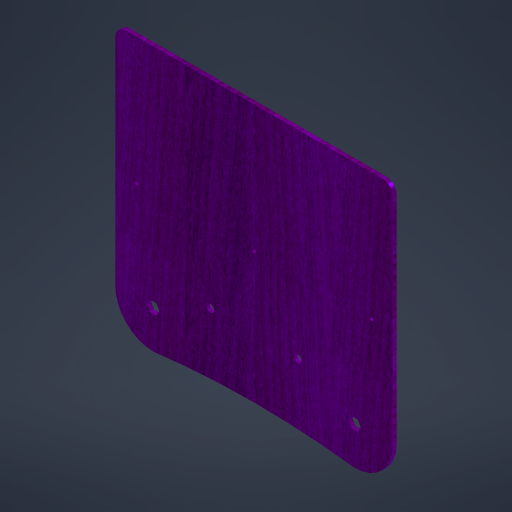
# Autodesk Inventor part: FTC Outside Panels
Saved by Autodesk Inventor 2024.2 (Build 282272000, 272)
## iProperties
Created: 2022-09-22
Part Number: FTC Outside Panels
Material: Wood (Oak)
Document SubType Name: Modeling
Designer: Jason
Density: 0.76 g/cm^3
Appearance: White Oak - Natural Medium Gloss
Author: Jason
Autodesk Inventor part; units mm, degrees
ref_plane "YZ Plane" through (0, 0, 0) normal (1, 0, 0) x (0, 1, 0)
ref_plane "XZ Plane" through (0, 0, 0) normal (0, 1, 0) x (-1, 0, 0)
ref_plane "XY Plane" through (0, 0, 0) normal (0, 0, 1) x (1, 0, 0)
sketch "Sketch1" plane through (0, 0, 0) normal (0, 0, 1) x (1, 0, 0)
  line L0 (0, 0) -> (333.375, 0)
  line L1 (333.375, 0) -> (333.375, 304.8)
  line L2 (320.675, 317.5) -> (12.7, 317.5)
  line L3 (0, 304.8) -> (0, 0)
  circle A0 centre (45.72, 45.72) radius 45.72
  circle A1 centre (287.655, 45.72) radius 45.72
  line L4 (166.6875, 0) -> (166.6875, 7.62)
  arc A2 (287.655, 0) -> (45.72, 0) centre (166.6875, -956.3695) ccw
  arc A3 (12.7, 317.5) -> (0, 304.8) centre (12.7, 304.8) ccw
  arc A4 (333.375, 304.8) -> (320.675, 317.5) centre (320.675, 304.8) ccw
  circle A5 centre (45.72, 45.72) radius 2.413
  circle A6 centre (287.655, 45.72) radius 2.413
  circle A7 centre (25.4, 165.1) radius 2.413
  circle A8 centre (307.975, 165.1) radius 2.413
  line L5 (25.4, 165.1) -> (307.975, 165.1)
  circle A9 centre (166.6875, 165.1) radius 2.413
  line L6 (114.0968, 95.337) -> (114.0968, 63.3371)
  line L7 (114.0968, 45.72) -> (114.0968, 63.3371)
  circle A10 centre (114.1277, 79.3382) radius 4.699
  ellipse E0 centre (114.0968, 63.3371) end of major axis (114.0894, 65.3371) minor radius 2
  line L8 (219.2782, 45.72) -> (219.2782, 63.3371)
  ellipse E1 centre (219.2782, 63.3371) end of major axis (219.2708, 65.3371) minor radius 2
  line L9 (219.2782, 95.3392) -> (219.2782, 63.3371)
  circle A11 centre (219.3091, 79.3382) radius 4.699
  line L10 (45.72, 45.72) -> (114.0968, 45.72)
  line L11 (287.655, 45.72) -> (219.2782, 45.72)
  ellipse E2 centre (235.2526, 141.4087) end of major axis (235.2552, 140.0562) minor radius 1.3525
  ellipse E3 centre (203.2527, 141.3472) end of major axis (203.2553, 139.9947) minor radius 1.3525
  ellipse E4 centre (219.2782, 95.3392) end of major axis (219.2743, 97.3392) minor radius 2
  ellipse E5 centre (219.2782, 95.3392) end of major axis (219.2743, 97.3392) minor radius 2
  ellipse E6 centre (130.4933, 141.0351) end of major axis (130.4959, 139.6826) minor radius 1.3525
  ellipse E7 centre (98.4934, 140.9736) end of major axis (98.496, 139.621) minor radius 1.3525
  ellipse E8 centre (114.0968, 95.337) end of major axis (114.0929, 97.337) minor radius 2
  ellipse E9 centre (114.0968, 95.337) end of major axis (114.0929, 97.337) minor radius 2
  line L12 (49.3862, 39.37) -> (53.0523, 45.72)
  line L13 (49.3862, 52.07) -> (53.0523, 45.72)
  line L14 (42.0538, 39.37) -> (49.3862, 39.37)
  line L15 (42.0538, 52.07) -> (49.3862, 52.07)
  line L16 (42.0538, 52.07) -> (38.3877, 45.72)
  line L17 (38.3877, 45.72) -> (42.0538, 39.37)
  line L18 (291.1818, 39.37) -> (294.848, 45.72)
  line L19 (291.1818, 52.07) -> (294.848, 45.72)
  line L20 (283.8495, 39.37) -> (291.1818, 39.37)
  line L21 (283.8495, 52.07) -> (291.1818, 52.07)
  line L22 (283.8495, 52.07) -> (280.1833, 45.72)
  line L23 (280.1833, 45.72) -> (283.8495, 39.37)
  line L24 (42.0538, 52.07) -> (49.3862, 39.37)
  line L25 (42.0538, 39.37) -> (49.3862, 52.07)
  point P0 (333.375, 317.5)
  point P1 (0, 317.5)
  point P2 (0, 0)
  point P3 (333.375, 45.72)
  point P4 (0, 45.72)
  point P5 (45.3639, 35.0229)
  point P6 (45.3639, 35.0229)
  point P7 (287.655, 45.72)
  point P8 (287.655, 45.72)
  point P9 (49.2468, 52.07)
  point P10 (291.1818, 52.07)
  point P11 (49.7423, 75.4671)
  point P12 (291.1818, 64.77)
  point P13 (45.72, 45.72)
  dimension "d176" = 91.44
  dimension "d177" = 91.44
  dimension "d174" = 333.375
  dimension "d175" = 317.5
  dimension "d178" = 7.62
  dimension "d179" = 12.7
  dimension "d180" = 4.826
  dimension "d181" = 4.826
  dimension "d182" = 4.826
  dimension "d184" = 25.4
  dimension "d185" = 4.826
  dimension "d186" = 25.4
  dimension "d188" = 4.826
  dimension "d189" = 17.6171
  dimension "d190" = 17.6171
  dimension "d191" = 9.398
  dimension "d192" = 9.398
  dimension "d193" = 68.3768
  dimension "d194" = 68.3768
  dimension "d195" = 165.1
  dimension "d206" = 12.7
  dimension "d207" = 12.7
  dimension "d208" = 12.7
  dimension "d209" = 7.3323
  dimension "d210" = 7.3323
  dimension "d211" = 7.3323
  dimension "d212" = 7.3323
  dimension "d213" = 7.3323
  dimension "d214" = 7.3323
  dimension "d215" = 12.7
  dimension "d216" = 12.7
  dimension "d217" = 12.7
  dimension "d218" = 7.3323
  dimension "d219" = 7.3323
  dimension "d220" = 7.3323
  dimension "d221" = 7.3323
  dimension "d222" = 7.3323
  dimension "d223" = 7.3323
  constraints: 52 end point, 14 centre point, 9 horizontal, 7 point on circle, 6 point on line, 6 vertical, 4 tangent, 3 midpoint, 2 coincident, 2 parallel, 1 equal radius, 1 perpendicular, 18 other
  measures "d174" distance of point (0, 317.5) point (333.375, 317.5)
  measures "d175" distance of point (333.375, 317.5) L0.end
  measures "d178" distance of L4.start L4.end
  measures "d179" radius of A3
  measures "d180" diameter of A5
  measures "d181" diameter of A6
  measures "d182" diameter of A7
  measures "d184" distance from line of L3 L5.start
  measures "d185" diameter of A8
  measures "d186" distance from line of L1 L5.end
  measures "d188" diameter of A9
  measures "d189" distance of L8.start L8.end
  measures "d190" distance of L7.start L7.end
  measures "d191" diameter of A11
  measures "d192" diameter of A10
  measures "d193" distance of L10.start L10.end
  measures "d194" distance of L11.start L11.end
  measures "d195" distance between parallel lines of L0 L5
  measures "d206" distance between parallel lines of L13 L17
  measures "d207" distance between parallel lines of L16 L12
  measures "d208" distance between parallel lines of L15 L14
  measures "d209" distance of L16.start L17.start
  measures "d210" distance of L17.start L14.start
  measures "d211" distance of L12.start L12.end
  measures "d212" distance of L14.start L12.start
  measures "d213" distance of L13.start L12.end
  measures "d214" distance of L16.start L15.end
  measures "d215" distance between parallel lines of L19 L23
  measures "d216" distance between parallel lines of L22 L18
  measures "d217" distance between parallel lines of L21 L20
  measures "d218" distance of L22.start L22.end
  measures "d219" distance of L22.end L23.end
  measures "d220" distance of L20.end L19.end
  measures "d221" distance of L23.end L20.end
  measures "d222" distance of L19.start L19.end
  measures "d223" distance of L22.start L21.end
extrude "Extrusion1" add sketch "Sketch1" along normal blind 4.699 contours A0 A2 | L3 A3 L2 A4 L1 A1 A2 A0 | A2 A1 | E0 L7 L6 | L6 L7 E0 | E1 L9 L8 | L8 L9 E1 | E2 | E3 | E4 | E6 | E7 | E8 picked at (16.5244, 31.421) picked at (316.8042, 60.019)
body "Solid1"
